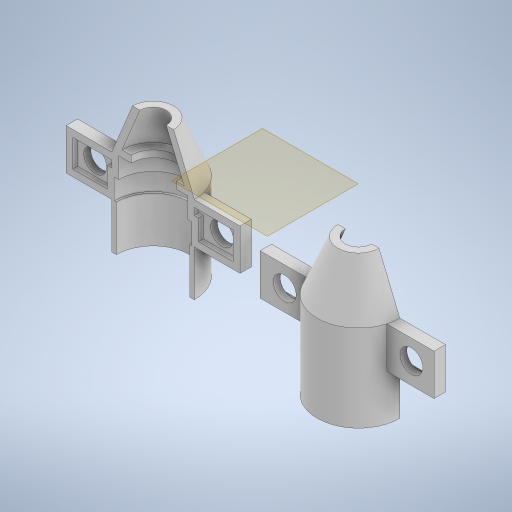
# Autodesk Inventor part: inner Part of male
Saved by Autodesk Inventor 2023 (Build 270158000, 158)
## iProperties
Created: 2022-10-17
Part Number: inner Part of male
Material: Generic
Document SubType Name: Modeling
Designer: rayle
Density: 1 g/cm^3
Appearance: Default
Author: rayle
Autodesk Inventor part; units mm, degrees
ref_plane "YZ Plane" through (0, 0, 0) normal (1, 0, 0) x (0, 1, 0)
ref_plane "XY Plane" through (0, 0, 0) normal (0, 0, 1) x (1, 0, 0)
sketch "Sketch1" plane through (0, 0, 0) normal (0, 1, 0) x (-1, 0, 0)
  line L0 (10.054, 0) -> (10.054, -1.53)
  line L1 (10.054, -1.53) -> (8.9238, -1.53)
  line L2 (10.054, 0) -> (10.054, 1.53)
  line L3 (10.054, 1.53) -> (8.9238, 1.53)
  arc A0 (8.9238, 1.53) -> (8.9238, -1.53) centre (0, 0) ccw
  circle A1 centre (0, 0) radius 8.05
  point P0 (0, 0)
  point P1 (2.5, -8.702)
  point P2 (-2.5, -8.702)
  point P3 (2.5, 8.702)
  point P4 (-2.5, 8.702)
  dimension "d3" = 1.53
  dimension "d65" = 16.1
  dimension "d69" = 9.054
  constraints: 8 end point, 6 point on circle, 2 centre point, 2 perpendicular, 1 coincident, 1 vertical
  measures "d3" distance of L0.start L0.end
  measures "d65" diameter of A1
  measures "d69" radius of A0
extrude "Extrusion1" add sketch "Sketch1" along normal blind 10
sketch "Sketch2" plane through (0, 10, 0) normal (0, 1, 0) x (1, 0, 0)
  circle A0 centre (0, 0) radius 9.054
  arc A1 (-8.9238, -1.53) -> (-8.9238, 1.53) centre (0, 0) ccw projected
  line L0 (0, 19.054) -> (2.5, 19.054)
  line L1 (2.5, 19.054) -> (2.5, 8.702)
  line L2 (0, 19.054) -> (-2.5, 19.054)
  line L3 (-2.5, 19.054) -> (-2.5, 8.702)
  line L4 (0, -19.054) -> (2.5, -19.054)
  line L5 (2.5, -19.054) -> (2.5, -8.702)
  line L6 (0, -19.054) -> (-2.5, -19.054)
  line L7 (-2.5, -19.054) -> (-2.5, -8.702)
  circle A2 centre (0, 0) radius 8.05 projected
  line L8 (0, 0) -> (-7.35, 0)
  circle A3 centre (0, 0) radius 8.5
  line L9 (-8.25, 2) -> (-8.389, 2)
  line L10 (-8.25, -2) -> (-8.2614, -2)
  line L11 (8.5, 0) -> (7.35, 0)
  line L12 (7.35, 0) -> (7.35, 2)
  line L13 (7.35, 2) -> (8.5, 2)
  line L14 (7.35, 0) -> (7.35, -2)
  line L15 (7.35, -2) -> (8.5, -2)
  point P0 (2.5, -8.702)
  point P1 (-2.5, -8.702)
  point P2 (-8.2614, 2)
  point P3 (8.2614, -2)
  point P4 (8.2614, 2)
  dimension "d45" = 2.5
  dimension "d46" = 2.5
  dimension "d48" = 2.5
  dimension "d49" = 2.5
  dimension "d70" = 17
  dimension "d71" = 1.15
  dimension "d73" = 2
  dimension "d74" = 2
  constraints: 32 end point, 7 horizontal, 6 point on circle, 5 perpendicular, 2 centre point, 2 vertical, 1 coincident
  measures "d45" distance of L0.start L0.end
  measures "d46" distance of L0.start L2.end
  measures "d48" distance of L4.start L4.end
  measures "d49" distance of L4.start L6.end
  measures "d70" diameter of A3
  measures "d71" distance of L11.start L11.end
  measures "d73" distance of L11.end L12.end
  measures "d74" distance of L11.end L14.end
extrude "Extrusion2" add sketch "Sketch2" along normal blind 4.5 contours A0 | A0 L3 L2 L0 L1 | L5 L4 L6 L7 A0 | L11 L12 L13 A2 | L11 A3 L15 A2 | A2 L13 A3 L11 | A2 L15 L14 L11
sketch "Sketch3" plane through (0, 14.5, 0) normal (0, 1, 0) x (0, 0, 1)
  circle A0 centre (0, 0) radius 9.054
  arc A1 (-8.702, 2.5) -> (-8.702, -2.5) centre (0, 0) ccw projected
  line L0 (-8.702, 2.5) -> (-19.054, 2.5) projected
  line L1 (-8.702, 2.5) -> (-19.054, 2.5)
  line L2 (-19.054, 2.5) -> (-19.054, -2.5) projected
  line L3 (-19.054, 2.5) -> (-19.054, -2.5)
  line L4 (-19.054, -2.5) -> (-8.702, -2.5)
  arc A2 (8.702, 2.5) -> (-8.702, 2.5) centre (0, 0) ccw projected
  line L5 (8.702, 2.5) -> (19.054, 2.5)
  line L6 (19.054, -2.5) -> (19.054, 2.5) projected
  line L7 (19.054, 2.5) -> (19.054, -2.5)
  line L8 (8.702, -2.5) -> (19.054, -2.5) projected
  line L9 (19.054, -2.5) -> (8.702, -2.5)
  circle A3 centre (0, 0) radius 7.55
  point P0 (19.054, 2.5)
  dimension "d103" = 15.1
  constraints: 12 end point, 2 centre point, 2 collinear, 2 perpendicular, 1 coincident, 1 horizontal, 1 point on circle
  measures "d103" diameter of A3
extrude "Extrusion3" add sketch "Sketch3" along normal blind 4.5
sketch "Sketch4" plane through (0, 19, 0) normal (0, 1, 0) x (0, 0, -1)
  circle A0 centre (0, 0) radius 9.054
  circle A1 centre (0, 0) radius 7.55
  constraints: 2 centre point, 2 coincident
ref_plane "Work Plane1" through (0, 30, 0) normal (0, 1, 0) x (-1, 0, 0)
sketch "Sketch10" plane through (0, 30, 0) normal (0, 1, 0) x (-1, 0, 0)
  circle A0 centre (0, 0) radius 4.5
  circle A1 centre (0, 0) radius 3.75
  dimension "d75" = 9
  dimension "d76" = 7.5
  constraints: 2 centre point, 2 coincident
  measures "d75" diameter of A0
  measures "d76" diameter of A1
loft "Loft3" add profiles "Sketch10", "Sketch4" contours A0 | A1 / A0 | A1
shell "Shell3" thickness 1.5 removed faces 1 at (-0.8473, 30, -0.3083)
sketch "Sketch15" plane through (-2.5, 10, -19.054) normal (-1, 0, 0) x (0, 0, 1)
  point P0 (19.054, -10)
  point P1 (4.9562, 4.6426)
hole "Hole8" at (-2.5, 14.6426, -14.0978) direction (1, 0, 0) diameter 5 depth 5 tip angle 118
sketch "Sketch16" plane through (-2.5, 10, 8.702) normal (-1, 0, 0) x (0, 0, 1)
  point P0 (-8.702, -10)
  point P1 (4.9609, 4.5701)
hole "Hole9" at (-2.5, 14.5701, 13.6629) direction (1, 0, 0) diameter 5 depth 5 tip angle 118
sketch "Sketch17" plane through (0, 20.5, 0) normal (0, 1, 0) x (1, 0, 0)
  point P0 (0, 0)
  point P1 (0.0501, 0.1611)
hole "Hole10" at (0.0501, 20.5, -0.1611) direction (0, -1, 0) diameter 10 depth 5 tip angle 118
split body "Split1" result two bodies by plane through (0, 0, 0) normal (1, 0, 0) first body at (0.953, 3.3333, -8.5008)
move or copy body "Move Body1" bodies to move or copy 2 copy no translate (10, 0, 0)
move or copy body "Move Body2" bodies to move or copy 2 copy no translate (10, 0, 0)
move or copy body "Move Body3" bodies to move or copy 3 copy no translate (-10, 0, 0)
move or copy body "Move Body4" bodies to move or copy 3 copy no rotation origin (0, 0, 0) rotation axis (0, 1, 0) rotation angle 90 translate (-10, 0, -10)
move or copy body "Move Body5" bodies to move or copy 2 copy no rotation origin (0, 0, 0) rotation axis (0, 1, 0) rotation angle -90 translate (20, 0, -20)
move or copy body "Move Body6" bodies to move or copy 3 copy no rotation origin (0, 0, 0) rotation axis (0, 1, 0) rotation angle 180 translate (-20, 0, 0)
move or copy body "Move Body7" bodies to move or copy 3 copy no translate (-15, 0, 0)
body "Solid2"
body "Solid3"
